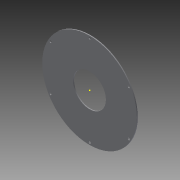
# Autodesk Inventor part: Base Plate
Saved by Autodesk Inventor 2016 (Build 200138000, 138)
## iProperties
Created: 2016-04-11
Part Number: Base Plate
Material: Generic
Document SubType Name: Modeling
Designer: rubenjm
Density: 1 g/cm^3
Appearance: Default
Author: rubenjm
Autodesk Inventor part; units mm, degrees
ref_plane "YZ Plane" through (0, 0, 0) normal (1, 0, 0) x (0, 1, 0)
ref_plane "XZ Plane" through (0, 0, 0) normal (0, 1, 0) x (-1, 0, 0)
ref_plane "XY Plane" through (0, 0, 0) normal (0, 0, 1) x (1, 0, 0)
sketch "Sketch1" plane through (0, 0, 0) normal (0, 0, 1) x (1, 0, 0)
  circle A0 centre (0, 0) radius 165.1
  circle A1 centre (0, 0) radius 57.15
  dimension "d0" = 330.2
  dimension "d3" = 114.3
  constraints: 2 centre point, 2 coincident
  measures "d0" diameter of A0
  measures "d3" diameter of A1
extrude "Extrusion2" add sketch "Sketch1" along normal blind 3.175
sketch "Sketch2" plane through (0, 0, 3.175) normal (0, 0, 1) x (1, 0, 0)
  point P0 (0, 0)
sketch "Sketch3" plane through (0, 0, 3.175) normal (0, 0, 1) x (1, 0, 0)
  circle A0 centre (0, 0) radius 157.48 construction
  circle A1 centre (0, 157.48) radius 3.9687
  circle A2 centre (-136.3817, 78.74) radius 3.9687
  circle A3 centre (-136.3817, -78.74) radius 3.9687
  circle A4 centre (0, -157.48) radius 3.9687
  circle A5 centre (136.3817, -78.74) radius 3.9687
  circle A6 centre (136.3817, 78.74) radius 3.9687
  dimension "d6" = 314.96
  dimension "d7" = 7.9375
  dimension "d10" = 360
  constraints: 6 centre point, 1 coincident, 1 vertical alignment, 15 other
  measures "d7" diameter of A1
extrude "Extrusion3" cut sketch "Sketch3" against normal through all
body "Solid2"
